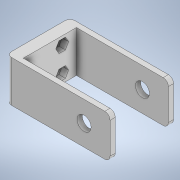
# Autodesk Inventor part: gfdsgfd
Saved by Autodesk Inventor 2022 (Build 260153000, 153)
## iProperties
Created: 2022-04-02
Part Number: gfdsgfd
Material: Genérico
Document SubType Name: Modeling
Designer: JK
Density: 1 g/cm^3
Appearance: Valor por defecto
Author: JK
Autodesk Inventor part; units mm, degrees
ref_plane "YZ Plane" through (0, 0, 0) normal (1, 0, 0) x (0, 1, 0)
ref_plane "XZ Plane" through (0, 0, 0) normal (0, 1, 0) x (-1, 0, 0)
ref_plane "XY Plane" through (0, 0, 0) normal (0, 0, 1) x (1, 0, 0)
sketch "Boceto1" plane through (0, 0, 0) normal (0, 1, 0) x (-1, 0, 0)
  line L0 (-10.7233, 10.25) -> (10.7233, 10.25)
  line L1 (10.7233, 10.25) -> (10.7233, -10.25)
  line L2 (10.7233, -10.25) -> (-10.7233, -10.25)
  line L3 (-10.7233, -10.25) -> (-10.7233, 10.25)
  line L4 (-10.7233, 10.25) -> (10.7233, -10.25) construction
  line L5 (10.7233, 10.25) -> (-10.7233, -10.25) construction
  line L6 (-10.7233, 12.25) -> (10.7233, 12.25)
  line L7 (10.7233, 12.25) -> (10.7233, -12.25)
  line L8 (10.7233, -12.25) -> (-10.7233, -12.25)
  line L9 (-10.7233, -12.25) -> (-10.7233, 12.25)
  line L10 (-10.7233, 12.25) -> (10.7233, -12.25) construction
  line L11 (10.7233, 12.25) -> (-10.7233, -12.25) construction
  line L12 (10.7233, 12.25) -> (24.7233, 12.25)
  line L13 (24.7233, 12.25) -> (24.7233, -12.25)
  line L14 (24.7233, -12.25) -> (10.7233, -12.25)
  line L15 (10.7233, -12.25) -> (10.7233, 12.25)
  line L16 (10.7233, 10.25) -> (24.7233, 10.25)
  line L17 (24.7233, 10.25) -> (24.7233, -10.25)
  line L18 (24.7233, -10.25) -> (10.7233, -10.25)
  line L19 (10.7233, -10.25) -> (10.7233, 10.25)
  line L20 (24.7233, 12.25) -> (29.2233, 12.25)
  line L21 (29.2233, 12.25) -> (29.2233, -12.25)
  line L22 (29.2233, -12.25) -> (24.7233, -12.25)
  line L23 (24.7233, -12.25) -> (24.7233, 12.25)
  point P0 (0, 0)
  point P1 (24.7233, 10.25)
  point P2 (-10.7233, -10.25)
  dimension "d0" = 20.5
  dimension "d1" = 2
  dimension "d2" = 14
  dimension "d3" = 18.5
  constraints: 48 end point, 10 parallel, 5 horizontal, 5 perpendicular, 4 midpoint, 2 collinear
  measures "d0" distance between parallel lines of L2 L0
  measures "d1" distance between parallel lines of L0 L6
  measures "d2" distance between parallel lines of L13 L1
  measures "d3" distance between parallel lines of L21 L1
extrude "Extrusión1" add sketch "Boceto1" along normal blind 16 contours L9 L6 L7 L0 | L7 L12 L13 L16 | L2 L7 L8 L9 | L18 L13 L14 L7 | L13 L20 L21 L22
sketch "Boceto2" plane through (-29.2233, 0, -12.25) normal (-1, 0, 0) x (0, 0, 1)
  circle A0 centre (7.5, 3.3) radius 1.15
  circle A1 centre (7.5, 12.8) radius 1.15
  line L0 (0, 0) -> (24.5, 0) projected
  line L1 (0, 0) -> (0, 16) projected
  point P0 (12.25, 0)
  dimension "d6" = 2.3
  dimension "d7" = 3.3
  dimension "d8" = 9.5
  dimension "d9" = 7.5
  constraints: 2 centre point, 1 equal radius, 1 vertical alignment
  measures "d6" diameter of A0
  measures "d7" distance from line of L0 A0.centre
  measures "d8" distance of A1.centre A0.centre
  measures "d9" distance from line of L1 A0.centre
extrude "Extrusión2" cut sketch "Boceto2" against normal through all
sketch "Boceto3" plane through (-24.7233, 0, 10.25) normal (1, 0, 0) x (0, 0, -1)
  circle A0 centre (15, 12.8) radius 1.15 projected
  circle A1 centre (15, 12.8) radius 2.15
  circle A2 centre (15, 3.3) radius 1.15 projected
  circle A3 centre (15, 3.3) radius 2.15
  line L0 (17.4826, 12.8) -> (16.2413, 10.65)
  line L1 (16.2413, 10.65) -> (13.7587, 10.65)
  line L2 (13.7587, 10.65) -> (12.5174, 12.8)
  line L3 (12.5174, 12.8) -> (13.7587, 14.95)
  line L4 (13.7587, 14.95) -> (16.2413, 14.95)
  line L5 (16.2413, 14.95) -> (17.4826, 12.8)
  line L6 (17.4826, 3.3) -> (16.2413, 1.15)
  line L7 (16.2413, 1.15) -> (13.7587, 1.15)
  line L8 (13.7587, 1.15) -> (12.5174, 3.3)
  line L9 (12.5174, 3.3) -> (13.7587, 5.45)
  line L10 (13.7587, 5.45) -> (16.2413, 5.45)
  line L11 (16.2413, 5.45) -> (17.4826, 3.3)
  point P0 (10.25, 0)
  dimension "d12" = 4.3
  constraints: 24 end point, 4 coincident, 2 centre point, 2 horizontal, 2 tangent, 1 equal radius, 26 other
  measures "d12" diameter of A1
extrude "Extrusión3" cut sketch "Boceto3" against normal blind 2.5 contours A0 | A1 | A1 L5 L0 | A1 L4 L5 | L0 L1 A1 | A1 L3 L4 | L1 L2 A1 | A1 L2 L3 | A2 | A3 | A3 L11 L6 | A3 L10 L11 | L6 L7 A3 | A3 L9 L10 | L7 L8 A3 | A3 L8 L9
sketch "Boceto4" plane through (-29.2233, 0, 12.25) normal (0, 0, 1) x (1, 0, 0)
  circle A0 centre (29.9467, 8) radius 2.7
  line L0 (39.9467, 0) -> (39.9467, 16) projected
  line L1 (0, 0) -> (39.9467, 0) projected
  point P0 (29.2233, 0)
  dimension "d15" = 10
  dimension "d16" = 8
  dimension "d17" = 5.4
  constraints: 1 centre point
  measures "d15" distance from line of A0.centre L0
  measures "d16" distance from line of L1 A0.centre
  measures "d17" diameter of A0
extrude "Extrusión4" cut sketch "Boceto4" against normal through all
fillet "Empalme1" radius 2 6 edges at (10.7233, 0, 11.25) (10.7233, 16, 11.25) (10.7233, 16, -11.25) (10.7233, 0, -11.25) (-29.2233, 8, 12.25) (-29.2233, 8, -12.25)
